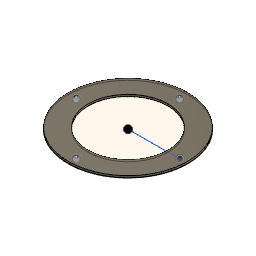
_platesensor.ecb4e9c5-dacc-4da2-a371-615c9f19e751 (Autodesk Fusion 360 design; units mm, degrees)
Autodesk Fusion 360 part; units mm, degrees
sketch "Sketch1" plane through (0, 0, 0) normal (0, 1, 0) x (1, 0, 0)
  circle A0 centre (0, 0) radius 60
  circle A1 centre (0, 0) radius 90
  circle A2 centre (78, 0.0519) radius 1.95
  line L0 (78, 0.0519) -> (0, 0)
  circle A3 centre (-0.0519, 78) radius 1.95
  circle A4 centre (-78, -0.0519) radius 1.95
  circle A5 centre (0.0519, -78) radius 1.95
  dimension "d1" = 120
  dimension "d2" = 180
  dimension "d3" = 3.9
  dimension "d4" = 78
  dimension "d6" = 360
  measures "d1" diameter of A0
  measures "d2" diameter of A1
  measures "d3" diameter of A2
  measures "d4" distance of A2.centre A0.centre
extrude "Extrude1" add sketch "Sketch1" along normal blind 3
